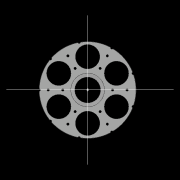
# Autodesk Inventor part: Top_Rotor_TSB
Saved by Autodesk Inventor 2022.2 (Build 262287010, 287A)
## iProperties
Created: 2022-05-21
Part Number: Top_Rotor_TSB
Material: Generic
Document SubType Name: Modeling
Designer: Árni Þór Þorgeirsson
Density: 1 g/cm^3
Appearance: Default
Author: Árni Þór Þorgeirsson
Autodesk Inventor part; units mm, degrees
ref_plane "YZ Plane" through (0, 0, 0) normal (1, 0, 0) x (0, 1, 0)
sketch "Sketch1" plane through (0, 0, 0) normal (0, 0, 1) x (1, 0, 0)
  circle A0 centre (0, 0) radius 13.3368 construction
  line L0 (0, 0) -> (13.3368, 0)
  line L1 (0, 0) -> (13.3368, 4.025)
  line L2 (13.3368, 0) -> (13.3368, 4.025)
  circle A1 centre (0, 0) radius 53.5
  dimension "d56" = 13.3368
  dimension "d57" = 4.025
  dimension "d400" = 53.5
  constraints: 6 end point, 2 coincident, 1 centre point, 1 horizontal, 1 horizontal alignment, 1 vertical, 6 other
  measures "d56" distance of L0.start L0.end
  measures "d57" distance of L1.end L0.end
  measures "d400" radius of A1
sketch "Sketch7" plane through (0, 0, 0) normal (0, 1, 0) x (-1, 0, 0)
  line L0 (0, 0) -> (0, 15.7673)
  line L1 (0, 0) -> (-13.3368, 0) construction
  line L2 (0, 15.7673) -> (-13.3368, 0) construction
  line L3 (0, 15.7673) -> (-18.6413, 0) construction
  line L4 (0, 15.7673) -> (-12.4569, -5.231) construction
  line L5 (0, 0) -> (0, -15.7673)
  line L6 (0, -15.7673) -> (-13.3368, 0) construction
  line L7 (0, -15.7673) -> (-18.6413, 0) construction
  line L8 (0, -15.7673) -> (-12.4569, 5.231) construction
  line L9 (-12.4569, 5.231) -> (-18.6413, 0) construction
  line L10 (-9.3537, 0) -> (-18.5948, -7.8164) construction
  line L11 (-9.3537, 0) -> (-18.0926, 7.3915) construction
  line L12 (0, -76.8701) -> (0, 74.6036) projected
  line L13 (-53.5, -5.9919) -> (-53.5, 6.008)
  line L14 (104.1947, 0) -> (-109.4074, 0) projected
  line L15 (-15.989, 2.2434) -> (-10.6846, -2.2434) construction
  line L16 (-10.6846, 2.2434) -> (-15.989, -2.2434) construction
  line L17 (-26.151, -15.9303) -> (-40.3783, -15.9303) construction
  line L18 (-40.3783, -15.9303) -> (-40.3783, -12.7539) construction
  line L19 (-40.3783, -12.7539) -> (-26.151, -12.7539) construction
  line L20 (-26.151, -12.7539) -> (-26.151, -15.9303) construction
  point P0 (-53.5, 0)
  dimension "Roller_Side_difference" = -0.0003
  dimension "d90" = 15.7673
  dimension "d201" = 53.5
  dimension "d343" = 99.548
  dimension "d344" = 99.549
  dimension "d367" = 8.1
  constraints: 28 end point, 9 point on line, 3 midpoint, 3 vertical, 2 horizontal, 2 parallel, 2 perpendicular, 1 collinear, 1 symmetric about line, 2 other
  measures "d90" distance of L0.start L0.end
  measures "d201" distance between parallel lines of L5 L13
  measures "d343" angle of L10 L8
  measures "d344" angle of L7 L10
  measures "d367" distance of L3.end L8.end
sketch "Roller1" plane through (0, 0, 0) normal (0, 1, 0) x (-1, 0, 0)
  line L0 (0, 15.7673) -> (-12.4569, -5.231) construction
  line L1 (0, 15.7673) -> (-18.6413, 0) construction
  line L2 (-9.3537, 0) -> (-18.0926, 7.3915) construction
  line L3 (0, -15.7673) -> (-18.6413, 0) construction
  line L4 (-9.4248, -0.0708) -> (-12.4245, -5.1274)
  line L5 (-12.4245, -5.1274) -> (-18.5445, 0.0491)
  line L6 (-18.5445, 0.0491) -> (-14.0556, 3.846)
  line L7 (-14.0556, 3.846) -> (-9.4248, -0.0708)
  line L8 (-11.7456, 1.8921) -> (-15.4898, -2.5346)
  line L9 (-10.9821, 1.2463) -> (-14.7263, -3.1804)
  point P0 (0, 0)
  point P1 (-15.4845, -2.5391)
  dimension "d345" = 0.025
  dimension "d346" = 0.025
  dimension "d347" = 0.1
  dimension "d348" = 0.1
  dimension "d349" = 99.549
  dimension "d350" = 99.548
  dimension "d357" = 1
  dimension "d369" = 4.0148
  constraints: 12 end point, 5 parallel, 4 point on line, 1 midpoint, 1 perpendicular
  measures "d345" distance between parallel lines of L0 L4
  measures "d346" distance between parallel lines of L1 L6
  measures "d347" distance between parallel lines of L3 L5
  measures "d348" distance between parallel lines of L2 L7
  measures "d349" angle of L6 L7
  measures "d350" angle of L4 L7
  measures "d357" distance between parallel lines of L8 L9
  measures "d369" distance from line of L4.end L8
sketch "Roller2" plane through (0, 0, 0) normal (0, 1, 0) x (-1, 0, 0)
  line L0 (0, -15.7673) -> (-12.4569, 5.231) construction
  line L1 (-9.3537, 0) -> (-18.5948, -7.8164) construction
  line L2 (0, -15.7673) -> (-18.6413, 0) construction
  line L3 (0, 15.7673) -> (-18.6413, 0) construction
  line L4 (-12.4633, 5.1928) -> (-9.386, 0.0054)
  line L5 (-9.386, 0.0054) -> (-13.9975, -3.8951)
  line L6 (-13.9975, -3.8951) -> (-18.6026, 0)
  line L7 (-18.6026, 0) -> (-12.4633, 5.1928)
  line L8 (-15.533, 2.5964) -> (-11.6918, -1.9449)
  line L9 (-14.7694, 3.2422) -> (-10.9283, -1.2991)
  point P0 (0, 0)
  dimension "d351" = 0.025
  dimension "d352" = 0.025
  dimension "d354" = 0.025
  dimension "d355" = 99.548
  dimension "d356" = 99.549
  dimension "d370" = 0.025
  dimension "d371" = 1
  constraints: 12 end point, 5 parallel, 3 point on line, 1 midpoint, 1 perpendicular
  measures "d351" distance between parallel lines of L0 L4
  measures "d352" distance between parallel lines of L2 L6
  measures "d354" distance between parallel lines of L1 L5
  measures "d355" angle of L5 L4
  measures "d356" angle of L6 L5
  measures "d370" distance from line of L3 L8.start
  measures "d371" distance between parallel lines of L9 L8
sketch "Sketch22" plane through (0, 0, 0) normal (0, 1, 0) x (-1, 0, 0)
  line L0 (-31.756, 8.0215) -> (-17.5287, 8.0215) construction
  line L1 (-17.5287, 8.0215) -> (-17.5287, 4.8451) construction
  line L2 (-17.5287, 4.8451) -> (-31.756, 4.8451) construction
  line L3 (-31.756, 4.8451) -> (-31.756, 8.0215) construction
  point P0 (0, 0)
  dimension "Roller_Side_difference" = -0.0003
  constraints: 2 other
sketch "Sketch2" plane through (0, 0, 0) normal (0, 1, 0) x (-1, 0, 0)
  line L0 (0, 0) -> (0, 13.3368) construction
  line L1 (0, 0) -> (-13.3368, 0) projected
  line L2 (0, 0) -> (0, -13.3368)
  line L3 (0, -13.3368) -> (-13.3368, 0) construction
  line L4 (0, 13.3368) -> (-13.3368, 0) construction
  line L5 (-78.8928, 52.9645) -> (0, 13.3368) construction
  line L6 (-34.8011, 15.91) -> (0, 13.3368) construction
  line L7 (-34.8011, 15.91) -> (0, -13.3368) construction
  line L8 (-48.3339, 16.9106) -> (0, -13.3368) construction
  point P0 (-17.4708, -4.134)
  constraints: 16 end point, 3 point on line, 1 perpendicular, 1 symmetric about line, 1 vertical
sketch "Sketch23" plane through (0, 0, 0) normal (0, 1, 0) x (-1, 0, 0)
  line L0 (0, -15.7673) -> (-12.4569, 5.231) construction
  line L1 (0, -15.7673) -> (-18.6413, 0) construction
  line L2 (0, 15.7673) -> (-12.4569, -5.231) construction
  line L3 (-12.4569, 5.231) -> (-18.6413, 0) construction
  line L4 (0, 15.7673) -> (-18.6413, 0) construction
  line L5 (-12.4569, 5.231) -> (-12.4569, -5.231) construction
  line L6 (104.1947, 0) -> (-109.4074, 0) projected
  line L7 (-11.538, 3.731) -> (-9.3549, 0.051)
  line L8 (-9.3549, -0.051) -> (-11.538, -3.731)
  line L9 (-14.269, 3.731) -> (-18.5898, 0.0764)
  line L10 (-18.5898, -0.0764) -> (-14.269, -3.731)
  arc A0 (-18.5898, 0.0764) -> (-18.5898, -0.0764) centre (-18.5252, 0) ccw
  arc A1 (-9.3549, -0.051) -> (-9.3549, 0.051) centre (-9.4409, 0) ccw
  line L11 (-11.538, 3.731) -> (-11.538, 5.231)
  line L12 (-11.538, 5.231) -> (-1, 5.231)
  line L13 (-1, 5.231) -> (-1, -5.231)
  line L14 (-1, -5.231) -> (-11.538, -5.231)
  line L15 (-11.538, -5.231) -> (-11.538, -3.731)
  line L16 (-14.269, 3.731) -> (-14.269, 5.231)
  line L17 (-14.269, 5.231) -> (-53.5, 5.231)
  line L18 (-53.5, 5.231) -> (-53.5, -5.231)
  line L19 (-14.269, -3.731) -> (-14.269, -5.231)
  line L20 (-14.269, -5.231) -> (-53.5, -5.231)
  line L21 (-12.4569, 5.231) -> (-12.4569, 5.231)
  line L22 (-12.4569, -5.231) -> (-12.4569, -5.231)
  line L23 (0, -76.8701) -> (0, 74.6036) projected
  line L24 (-18.68, 0) -> (-53.5, 0)
  point P0 (0, 0)
  point P1 (-9.3246, 0)
  point P2 (-18.6252, 0)
  point P3 (-53.5, 0)
  dimension "d378" = 90
  dimension "d379" = 0.1
  dimension "d380" = 0.025
  dimension "d381" = 0.025
  dimension "d382" = 0.025
  dimension "d383" = 0.025
  dimension "d384" = 10.4619
  dimension "d385" = 0
  dimension "d386" = 0
  dimension "d391" = 1
  dimension "d392" = 53.5
  dimension "d393" = 1.5
  dimension "d394" = 1.5
  dimension "d395" = 1.5
  dimension "d396" = 1.5
  constraints: 36 end point, 10 point on line, 9 vertical, 4 horizontal, 4 parallel, 4 point on circle, 4 tangent, 2 centre point, 1 equal radius, 1 midpoint
  measures "d378" angle of L6 L5
  measures "d379" radius of A0
  measures "d380" distance between parallel lines of L9 L4
  measures "d381" distance between parallel lines of L10 L1
  measures "d382" distance between parallel lines of L0 L7
  measures "d383" distance between parallel lines of L2 L8
  measures "d384" distance of L0.end L2.end
  measures "d385" distance of L2.end L22.end
  measures "d386" distance of L0.end L21.end
  measures "d391" distance between parallel lines of L23 L13
  measures "d392" distance between parallel lines of L18 L23
  measures "d393" distance of L9.start L16.end
  measures "d394" distance of L7.start L11.end
  measures "d395" distance of L14.end L8.end
  measures "d396" distance of L10.end L19.end
revolve "RevRoller1" [suppressed]
fillet "Fillet1" [suppressed]
pattern_circular "Circular Pattern13" [suppressed]
feature "Move Body7" [suppressed]
revolve "Revolution13" [suppressed]
fillet "Fillet3" [suppressed]
pattern_circular "Circular Pattern14" [suppressed]
feature "Move Body6" [suppressed]
revolve "Revolution14" [suppressed]
revolve "OuterRim_Top2" add sketch "Sketch23" angle 360 about axis through (0, 0, -10) along (0, 0, 1) contours L6 A0 L10 L19 L20 L18
revolve "OuterRim_Bottom2" [suppressed]
extrude "Rotor_Ring" [suppressed]
draft "FaceDraft2" angle 2.5 pull direction (0, 0, 1) faces at (-39.8716, -35.6721, -1.7437) fixed edges at (-53.5, 0, -5.231)
sketch "Sketch30" plane through (0, 0, 5.231) normal (0, 0, 1) x (1, 0, 0)
  circle A0 centre (0, 0) radius 1 projected
  line L0 (0, 0) -> (2.5, 0)
  circle A1 centre (2.5, 0) radius 4
  dimension "d495" = 2.5
  dimension "d496" = 8
  constraints: 2 end point, 1 centre point, 1 coincident, 1 horizontal
  measures "d495" distance of L0.start L0.end
  measures "d496" diameter of A1
ref_plane "Work Plane5" through (0, 0, 50) normal (0, 0, 1) x (1, 0, 0)
sketch "Rotor Featurs" plane through (0, 0, 50) normal (0, 0, 1) x (1, 0, 0)
  circle A0 centre (0, 0) radius 53.5 projected
  circle A1 centre (0, 0) radius 14.269 projected
  circle A2 centre (0, 0) radius 1 projected
  circle A3 centre (0, 0) radius 43.5
  circle A4 centre (0, 0) radius 36.75
  circle A5 centre (0, 0) radius 27.5
  line L0 (-56.25, 1.5877) -> (-53.5, 3.1754)
  line L1 (-53.5, 3.1754) -> (-50.75, 1.5877)
  line L2 (-50.75, 1.5877) -> (-50.75, -1.5877)
  line L3 (-50.75, -1.5877) -> (-53.5, -3.1754)
  line L4 (-53.5, -3.1754) -> (-56.25, -1.5877)
  line L5 (-56.25, -1.5877) -> (-56.25, 1.5877)
  line L6 (-40.75, -1.5877) -> (-43.5, -3.1754)
  line L7 (-43.5, -3.1754) -> (-46.25, -1.5877)
  line L8 (-46.25, -1.5877) -> (-46.25, 1.5877)
  line L9 (-46.25, 1.5877) -> (-43.5, 3.1754)
  line L10 (-43.5, 3.1754) -> (-40.75, 1.5877)
  line L11 (-40.75, 1.5877) -> (-40.75, -1.5877)
  line L12 (-30.25, 1.5877) -> (-27.5, 3.1754)
  line L13 (-27.5, 3.1754) -> (-24.75, 1.5877)
  line L14 (-24.75, 1.5877) -> (-24.75, -1.5877)
  line L15 (-24.75, -1.5877) -> (-27.5, -3.1754)
  line L16 (-27.5, -3.1754) -> (-30.25, -1.5877)
  line L17 (-30.25, -1.5877) -> (-30.25, 1.5877)
  circle A6 centre (-31.8264, -18.375) radius 13.5
  circle A7 centre (-53.5, 0) radius 1.5
  circle A8 centre (-53.5, 0) radius 2.75
  circle A9 centre (-43.5, 0) radius 1.5
  circle A10 centre (-27.5, 0) radius 1.5
  circle A11 centre (-43.5, 0) radius 2.75
  circle A12 centre (-27.5, 0) radius 2.75
  line L18 (-11.6213, -17.5209) -> (20.5249, -17.5209) construction
  line L19 (20.5249, -17.5209) -> (20.5249, -24.7583) construction
  line L20 (20.5249, -24.7583) -> (-11.6213, -24.7583) construction
  line L21 (-11.6213, -24.7583) -> (-11.6213, -17.5209) construction
  circle A13 centre (0, 0) radius 18.6252 projected
  line L22 (-56.25, 7.1754) -> (-50.75, 7.1754)
  line L23 (-50.75, 7.1754) -> (-50.75, 6.1754)
  line L24 (-50.75, 6.1754) -> (-56.25, 6.1754)
  line L25 (-56.25, 6.1754) -> (-56.25, 7.1754)
  line L26 (-56.25, -7.1754) -> (-56.25, -6.1754)
  line L27 (-56.25, -6.1754) -> (-50.75, -6.1754)
  line L28 (-50.75, -7.1754) -> (-56.25, -7.1754)
  line L29 (-50.75, -6.1754) -> (-50.75, -7.1754)
  point P0 (-56.25, -1.5877)
  point P1 (-50.75, -1.5877)
  dimension "d534" = 87
  dimension "d535" = 73.5
  dimension "d536" = 55
  dimension "Bearing_Roller_Gap_Reduction" = 0.3
  dimension "d531" = 5.5
  dimension "d532" = 5.5
  dimension "d533" = 5.5
  dimension "d537" = 27
  dimension "d538" = 3
  dimension "d543" = 5.5
  dimension "d549" = 3
  dimension "d550" = 3
  dimension "d567" = 5.5
  dimension "d568" = 5.5
  dimension "d617" = 1
  dimension "d618" = 3
  dimension "d621" = 360
  constraints: 52 end point, 12 coincident, 7 centre point, 4 point on line, 3 horizontal alignment, 2 parallel, 1 collinear, 1 horizontal, 1 perpendicular, 70 other
  measures "d531" distance between parallel lines of L5 L2
  measures "d532" distance between parallel lines of L11 L8
  measures "d533" distance between parallel lines of L17 L14
  measures "d537" diameter of A6
  measures "d538" diameter of A7
  measures "d543" diameter of A8
  measures "d549" diameter of A9
  measures "d550" diameter of A10
  measures "d567" diameter of A11
  measures "d568" diameter of A12
  measures "d617" distance of L22.end L23.end
  measures "d618" distance from line of L24 L0.end
sketch "RotorRim_Bottom" plane through (0, 0, 5.231) normal (0, 0, 1) x (1, 0, 0)
  line L0 (-53.5, 3.1754) -> (-50.75, 1.5877) projected
  line L1 (-56.25, 1.5877) -> (-53.5, 3.1754) projected
  line L2 (-56.25, -1.5877) -> (-56.25, 1.5877) projected
  line L3 (-53.5, -3.1754) -> (-56.25, -1.5877) projected
  line L4 (-50.75, -1.5877) -> (-53.5, -3.1754) projected
  circle A0 centre (0, 0) radius 53.5 projected
  circle A1 centre (-53.5, 0) radius 1.5 projected
  point P0 (-53.4088, 3.1228)
  point P1 (-53.4088, -3.1228)
  point P2 (-53.479, -1.4999)
  point P3 (-53.479, 1.4999)
  constraints: 1 other
extrude "Extrusion24" [suppressed]
extrude "Extrusion25" [suppressed]
sketch "Sketch40" plane through (0, 0, -5.231) normal (0, 0, -1) x (-1, 0, 0)
  circle A0 centre (53.5, 0) radius 2.75 projected
  circle A1 centre (0, 0) radius 53.5 projected
  point P0 (53.4293, 2.7491)
  point P1 (53.4293, -2.7491)
extrude "Extrusion26" [suppressed]
pattern_circular "Circular Pattern23" [suppressed]
sketch "Sketch41" plane through (0, 0, 5.231) normal (0, 0, 1) x (1, 0, 0)
  circle A0 centre (0, 0) radius 53.5 projected
  circle A1 centre (-53.5, 0) radius 1.5 projected
  circle A2 centre (-43.5, 0) radius 1.5 projected
  circle A3 centre (-27.5, 0) radius 1.5 projected
  line L0 (-53.5, 3.1754) -> (-50.75, 1.5877) projected
  line L1 (-50.75, 1.5877) -> (-50.75, -1.5877) projected
  line L2 (-50.75, -1.5877) -> (-53.5, -3.1754) projected
  line L3 (-46.25, 1.5877) -> (-43.5, 3.1754) projected
  line L4 (-46.25, -1.5877) -> (-46.25, 1.5877) projected
  line L5 (-43.5, -3.1754) -> (-46.25, -1.5877) projected
  line L6 (-40.75, -1.5877) -> (-43.5, -3.1754) projected
  line L7 (-40.75, 1.5877) -> (-40.75, -1.5877) projected
  line L8 (-43.5, 3.1754) -> (-40.75, 1.5877) projected
  line L9 (-30.25, 1.5877) -> (-27.5, 3.1754) projected
  line L10 (-30.25, -1.5877) -> (-30.25, 1.5877) projected
  line L11 (-27.5, -3.1754) -> (-30.25, -1.5877) projected
  line L12 (-24.75, -1.5877) -> (-27.5, -3.1754) projected
  line L13 (-24.75, 1.5877) -> (-24.75, -1.5877) projected
  line L14 (-27.5, 3.1754) -> (-24.75, 1.5877) projected
  circle A4 centre (-31.8264, -18.375) radius 13.5 projected
  point P0 (-53.4088, -3.1228)
  point P1 (-53.4088, 3.1228)
  point P2 (-53.479, 1.4999)
  point P3 (-53.479, -1.4999)
extrude "Extrusion27" [suppressed]
extrude "Extrusion28" [suppressed]
pattern_circular "Circular Pattern24" [suppressed]
extrude "Extrusion29" [suppressed]
extrude "Extrusion30" [suppressed]
extrude "Extrusion31" [suppressed]
pattern_of_nothing "Circular Pattern25"
sketch "Sketch42" plane through (0, 0, -5.231) normal (0, 0, -1) x (-1, 0, 0)
  circle A0 centre (53.5, 0) radius 2.75 projected
  circle A1 centre (0, 0) radius 53.5 projected
  circle A2 centre (43.5, 0) radius 2.75 projected
  circle A3 centre (27.5, 0) radius 2.75 projected
  circle A4 centre (53.5, 0) radius 1.5 projected
  circle A5 centre (43.5, 0) radius 1.5 projected
  circle A6 centre (27.5, 0) radius 1.5 projected
  circle A7 centre (31.8264, -18.375) radius 13.5 projected
  point P0 (53.4293, 2.7491)
  point P1 (53.4293, -2.7491)
  point P2 (53.479, 1.4999)
  point P3 (53.479, -1.4999)
extrude "Extrusion32" cut sketch "Sketch42" against normal blind 3 contours A1 A4 A0 | A1 A4 picked at (51.1832, -0.0597) picked at (53.0311, 0.3425)
extrude "Extrusion33" cut sketch "Sketch42" against normal blind 5.231 contours A1 A4 picked at (53.0311, 0.3425)
extrude "Extrusion34" cut sketch "Sketch42" against normal blind 3 contours A2 | A3 | A5 | A6
extrude "Extrusion35" cut sketch "Sketch42" against normal blind 5.231 contours A5 | A6 | A7
pattern_circular "Circular Pattern26" count 9 over 360 about axis through (0, 0, -10) along (0, 0, 1) of "Extrusion32", "Extrusion33"
pattern_circular "Circular Pattern27" count 6 over 360 about axis through (0, 0, -10) along (0, 0, 1) of "Extrusion34", "Extrusion35"
chamfer "Chamfer1" [suppressed]
chamfer "Chamfer2" [suppressed]
feature "FaceDraft4" [suppressed]
ref_plane "Work Plane7" through (-0.5825, 0.0099, -55.231) normal (0, 0, -1) x (-1, 0, 0)
sketch "Sketch44" plane through (-0.5825, 0.0099, -55.231) normal (0, 0, -1) x (-1, 0, 0)
  point P0 (58.7175, -0.0099)
sketch "Sketch45" plane through (0, 0, 50) normal (0, 0, 1) x (1, 0, 0)
  point P0 (-51.8, 0)
extrude "Extrusion39" cut sketch "Rotor Featurs" along normal blind 0.8 from surface at -55.231 contours L22 L23 L24 A0 | A0 L24 L25 L22 | L28 L26 L27 A0 | A0 L27 L29 L28
extrude "Extrusion40" [suppressed]
ref_plane "Work Plane8" through (0, 0, 20) normal (0, 0, 1) x (1, 0, 0)
sketch "Sketch46" plane through (0, 0, 20) normal (0, 0, 1) x (1, 0, 0)
  spline S0 degree 3 poles (56.8, 0) (56.8, -1.4319) (57.0266, -2.8218) (57.3141, -4.0377) (57.7676, -5.9558) (58.3249, -7.5697) (58.7222, -9.3953) (59.1369, -11.3012) (59.3869, -13.435) (59.2247, -15.7235) (59.0417, -18.3045) (58.3019, -21.0371) (57.0692, -23.4317) (55.9716, -25.5639) (54.5147, -27.4028) (52.9916, -28.8594) (51.6098, -30.1808) (50.1991, -31.1871) (48.7772, -32.1565) (47.6582, -32.9193) (46.4886, -33.6761) (45.2876, -34.7145) (44.2461, -35.6149) (43.2239, -36.7614) (42.4465, -37.9481) (41.5522, -39.3132) (40.9615, -40.6395) (40.4023, -41.8816) (39.6981, -43.4458) (39.012, -44.9714) (38.0364, -46.5419) (36.8523, -48.4481) (35.229, -50.3909) (33.1724, -51.9911) (31.0828, -53.6171) (28.5762, -54.8431) (26.0987, -55.5082) (23.9667, -56.0805) (21.8887, -56.2534) (19.9964, -56.2163) (18.2263, -56.1816) (16.6275, -55.9648) (14.8704, -55.8135) (13.6437, -55.7079) (12.287, -55.6403) (10.8418, -55.7977) (9.4051, -55.954) (7.9582, -56.3561) (6.723, -56.8409) (4.72, -57.6271) (3.1609, -58.5239) (1.3743, -59.2859) (-0.4339, -60.0571) (-2.4841, -60.7211) (-4.7859, -61.008) (-7.2974, -61.3212) (-10.0699, -61.1458) (-12.6364, -60.4279) (-15.0685, -59.7477) (-17.2767, -58.6047) (-19.0781, -57.3063) (-20.675, -56.1553) (-21.9478, -54.9116) (-23.1791, -53.6504) (-24.0931, -52.7142) (-25.0062, -51.7331) (-26.1738, -50.758) (-27.2513, -49.8582) (-28.5815, -49.0078) (-29.9203, -48.4225) (-31.362, -47.7921) (-32.7293, -47.438) (-34.0061, -47.1128) (-35.7099, -46.6787) (-37.3575, -46.2745) (-39.1066, -45.5849) (-41.1221, -44.7903) (-43.2458, -43.605) (-45.1448, -41.9571) (-47.1257, -40.238) (-48.8124, -38.0317) (-49.9482, -35.7294) (-50.9787, -33.6408) (-51.5623, -31.5143) (-51.8755, -29.5515) (-52.1638, -27.7446) (-52.2245, -26.087) (-52.3894, -24.2693) (-52.5001, -23.0492) (-52.6748, -21.7055) (-53.0824, -20.3178) (-53.486, -18.9435) (-54.1251, -17.6047) (-54.8078, -16.4847) (-55.8849, -14.7175) (-56.9946, -13.3786) (-58.0206, -11.8296) (-59.0577, -10.2638) (-60.0421, -8.4781) (-60.746, -6.3918) (-61.5632, -3.97) (-61.9524, -1.1678) (-61.7393, 1.5511) (-61.5477, 3.9947) (-60.8853, 6.3317) (-59.9849, 8.3224) (-59.1769, 10.1091) (-58.2036, 11.607) (-57.2044, 13.0158) (-56.3467, 14.2251) (-55.4319, 15.3943) (-54.5714, 16.8827) (-53.8946, 18.0531) (-53.296, 19.4496) (-52.9414, 20.8302) (-52.5526, 22.3437) (-52.4247, 23.7538) (-52.324, 25.055) (-52.1844, 26.8594) (-52.0852, 28.5763) (-51.715, 30.453) (-51.2878, 32.618) (-50.4834, 34.9703) (-49.1585, 37.1767) (-47.7999, 39.439) (-45.9031, 41.4933) (-43.8164, 43.0144) (-41.9871, 44.3479) (-40.05, 45.273) (-38.2187, 45.9151) (-36.4508, 46.5351) (-34.7962, 46.8888) (-33.0011, 47.3754) (-31.816, 47.6967) (-30.5213, 48.102) (-29.2246, 48.7472) (-27.9361, 49.3883) (-26.7251, 50.2594) (-25.7377, 51.1332) (-24.1248, 52.5605) (-22.9654, 53.9373) (-21.5425, 55.266) (-20.1382, 56.5772) (-18.4817, 57.8699) (-16.4757, 58.9115) (-14.1658, 60.1108) (-11.4118, 60.9217) (-8.673, 61.1141) (-6.2167, 61.2866) (-3.8151, 60.9744) (-1.7249, 60.3891) (0.129, 59.87) (1.7254, 59.1596) (3.276, 58.4164) (4.5061, 57.8267) (5.74, 57.1881) (7.2319, 56.649) (8.5094, 56.1873) (9.9929, 55.8479) (11.4103, 55.7465) (12.9863, 55.6336) (14.4057, 55.7628) (15.7204, 55.893) (17.5126, 56.0705) (19.2283, 56.2635) (21.1474, 56.213) (23.3514, 56.155) (25.8006, 55.7542) (28.1882, 54.8225) (30.6413, 53.8653) (32.9754, 52.3479) (34.8186, 50.5592) (36.4742, 48.9526) (37.7272, 47.1676) (38.6791, 45.4442) (39.6023, 43.7728) (40.2354, 42.1708) (41.0732, 40.4265) (41.6043, 39.3209) (42.257, 38.119) (43.1325, 36.9822) (43.9863, 35.8733) (45.0213, 34.896) (46.0149, 34.1163) (47.6582, 32.827) (49.1789, 31.938) (50.7017, 30.7916) (52.2598, 29.6185) (53.8446, 28.1841) (55.2311, 26.3515) (56.7985, 24.28) (58.0545, 21.7118) (58.7031, 19.0595) (59.2916, 16.6532) (59.3854, 14.2226) (59.1574, 12.0576) (58.9571, 10.1553) (58.5292, 8.4737) (58.0655, 6.8215) (57.7157, 5.5753) (57.3275, 4.3132) (57.063, 2.8386) (56.9031, 1.9472) (56.8, 0.9776) (56.8, 0) knots 0 0 0 0 3.630189 3.630189 3.630189 9.356968 9.356968 9.356968 15.335248 15.335248 15.335248 22.077576 22.077576 22.077576 28.081487 28.081487 28.081487 33.527934 33.527934 33.527934 37.813991 37.813991 37.813991 41.530754 41.530754 41.530754 45.806559 45.806559 45.806559 51.191166 51.191166 51.191166 57.726747 57.726747 57.726747 64.367473 64.367473 64.367473 70.081985 70.081985 70.081985 75.427611 75.427611 75.427611 79.15967 79.15967 79.15967 82.86972 82.86972 82.86972 88.885508 88.885508 88.885508 94.974003 94.974003 94.974003 101.617247 101.617247 101.617247 107.912495 107.912495 107.912495 113.492866 113.492866 113.492866 117.63499 117.63499 117.63499 121.457377 121.457377 121.457377 125.573774 125.573774 125.573774 131.06692 131.06692 131.06692 137.396362 137.396362 137.396362 143.99916 143.99916 143.99916 149.989436 149.989436 149.989436 155.503632 155.503632 155.503632 159.204798 159.204798 159.204798 162.870082 162.870082 162.870082 168.653221 168.653221 168.653221 174.498759 174.498759 174.498759 181.284424 181.284424 181.284424 187.383433 187.383433 187.383433 192.857431 192.857431 192.857431 197.5563 197.5563 197.5563 201.251307 201.251307 201.251307 205.301831 205.301831 205.301831 210.91873 210.91873 210.91873 217.398706 217.398706 217.398706 224.043346 224.043346 224.043346 229.86837 229.86837 229.86837 235.491984 235.491984 235.491984 239.204835 239.204835 239.204835 242.894294 242.894294 242.894294 248.920758 248.920758 248.920758 254.86843 254.86843 254.86843 261.717359 261.717359 261.717359 267.860024 267.860024 267.860024 273.30815 273.30815 273.30815 277.630663 277.630663 277.630663 281.332185 281.332185 281.332185 285.447681 285.447681 285.447681 291.057972 291.057972 291.057972 297.50109 297.50109 297.50109 304.120892 304.120892 304.120892 310.066772 310.066772 310.066772 315.832644 315.832644 315.832644 319.487459 319.487459 319.487459 323.052251 323.052251 323.052251 328.947474 328.947474 328.947474 334.97976 334.97976 334.97976 341.798889 341.798889 341.798889 347.985491 347.985491 347.985491 353.421408 353.421408 353.421408 357.521549 357.521549 357.521549 360 360 360 360 projected
  circle A0 centre (62.6801, -0.0744) radius 6
  line L0 (0, 0) -> (-2.5, 0)
  circle A1 centre (50.2755, 38.2517) radius 6
  circle A2 centre (17.7125, 61.9669) radius 6
  circle A3 centre (-22.571, 62.0129) radius 6
  circle A4 centre (-55.1881, 38.3721) radius 6
  circle A5 centre (-67.6801, 0.0744) radius 6
  circle A6 centre (-55.2755, -38.2517) radius 6
  circle A7 centre (-22.7125, -61.9669) radius 6
  circle A8 centre (17.571, -62.0129) radius 6
  circle A9 centre (50.1881, -38.3721) radius 6
  spline S1 degree 3 poles (56.8, 0) (56.8, -1.327) (57.0234, -2.6109) (57.3007, -3.6923) (57.7543, -5.4607) (58.2895, -6.8218) (58.7112, -8.3283) (59.1721, -9.9753) (59.5267, -11.7944) (59.5593, -13.8117) (59.598, -16.208) (59.1382, -18.8439) (58.1536, -21.2237) (57.2965, -23.2955) (56.0684, -25.1435) (54.7369, -26.6222) (53.5473, -27.9433) (52.3032, -28.9676) (51.052, -29.9022) (50.046, -30.6537) (49.006, -31.3468) (47.8554, -32.3233) (46.9843, -33.0626) (46.0484, -34.0152) (45.2938, -35.1119) (44.5396, -36.2079) (44.0054, -37.3704) (43.6138, -38.3974) (42.983, -40.052) (42.6128, -41.4454) (42.0619, -42.8993) (41.4492, -44.516) (40.6333, -46.2151) (39.4339, -47.8713) (38.032, -49.8072) (36.0969, -51.6271) (33.9087, -52.9343) (31.9495, -54.1046) (29.8285, -54.8554) (27.8576, -55.2437) (26.1429, -55.5815) (24.5642, -55.6603) (23.0139, -55.6752) (21.7466, -55.6873) (20.4668, -55.6358) (18.9158, -55.7787) (17.7446, -55.8866) (16.399, -56.1544) (15.1593, -56.6349) (13.9089, -57.1195) (12.8329, -57.7662) (11.9323, -58.3732) (10.4683, -59.3599) (9.3245, -60.279) (7.9625, -61.1406) (6.4559, -62.0937) (4.6989, -62.9801) (2.6661, -63.5673) (0.3544, -64.235) (-2.2833, -64.4684) (-4.7798, -64.1594) (-7.0414, -63.8794) (-9.1504, -63.1755) (-10.9222, -62.2948) (-12.4361, -61.5424) (-13.6962, -60.6844) (-14.941, -59.7881) (-15.9425, -59.067) (-16.9561, -58.2795) (-18.3098, -57.5157) (-19.3549, -56.926) (-20.6338, -56.3928) (-21.9035, -56.0972) (-23.2354, -55.7871) (-24.4767, -55.715) (-25.5637, -55.6914) (-27.252, -55.6547) (-28.7024, -55.7096) (-30.3012, -55.5868) (-32.1878, -55.4419) (-34.2662, -55.0517) (-36.3567, -54.2041) (-38.6022, -53.2938) (-40.805, -51.844) (-42.5524, -50.0858) (-44.1477, -48.4804) (-45.35, -46.659) (-46.1982, -44.9141) (-46.94, -43.3878) (-47.4157, -41.9455) (-47.9119, -40.4276) (-48.2662, -39.3437) (-48.6345, -38.1705) (-49.2732, -36.8659) (-49.8415, -35.7053) (-50.6735, -34.4812) (-51.5908, -33.5134) (-52.5793, -32.4705) (-53.5785, -31.7191) (-54.4815, -31.054) (-55.7719, -30.1035) (-56.9658, -29.2673) (-58.1708, -28.1834) (-59.6101, -26.8888) (-61.0408, -25.2456) (-62.1667, -23.2509) (-63.4169, -21.0357) (-64.2365, -18.4173) (-64.477, -15.9) (-64.6864, -13.708) (-64.4799, -11.6321) (-64.0824, -9.8109) (-63.7377, -8.2319) (-63.2593, -6.8589) (-62.7733, -5.3187) (-62.4416, -4.2676) (-62.0874, -3.086) (-61.9088, -1.6884) (-61.7416, -0.3793) (-61.7884, 1.0779) (-62.0061, 2.3332) (-62.2809, 3.918) (-62.7245, 5.173) (-63.1084, 6.3618) (-63.5857, 7.8398) (-64.0285, 9.2882) (-64.3004, 10.9509) (-64.6311, 12.9738) (-64.6775, 15.2937) (-64.2284, 17.6343) (-63.7598, 20.0763) (-62.7437, 22.4881) (-61.4161, 24.469) (-60.332, 26.0866) (-59.0714, 27.4119) (-57.8129, 28.4988) (-56.5938, 29.5517) (-55.3903, 30.3668) (-54.0597, 31.3676) (-53.2039, 32.0113) (-52.2562, 32.7675) (-51.3507, 33.7733) (-50.4416, 34.783) (-49.6557, 36.0299) (-49.1234, 37.1808) (-48.4221, 38.6971) (-48.0555, 40.0041) (-47.6412, 41.2524) (-47.15, 42.7324) (-46.6064, 44.2048) (-45.7763, 45.7355) (-44.7411, 47.6446) (-43.2412, 49.6031) (-41.3334, 51.2075) (-39.4289, 52.809) (-37.1526, 54.0167) (-34.9373, 54.7142) (-33.1141, 55.2883) (-31.3598, 55.5342) (-29.7323, 55.6242) (-28.3513, 55.7006) (-27.0633, 55.6597) (-25.5864, 55.6909) (-24.5244, 55.7133) (-23.3181, 55.7804) (-22.0174, 56.0712) (-20.725, 56.3602) (-19.4113, 56.8974) (-18.3415, 57.4978) (-16.8985, 58.3079) (-15.8405, 59.1437) (-14.7779, 59.9053) (-13.4787, 60.8365) (-12.1375, 61.7296) (-10.5152, 62.4916) (-8.5819, 63.3996) (-6.2624, 64.0777) (-3.8277, 64.2524) (-1.4092, 64.426) (1.0769, 64.0915) (3.2393, 63.3918) (5.2098, 62.7542) (6.8896, 61.8487) (8.3517, 60.8899) (9.6525, 60.0367) (10.7724, 59.1259) (12.2575, 58.1575) (13.172, 57.5612) (14.2777, 56.9407) (15.5201, 56.5012) (16.758, 56.0632) (18.0589, 55.8429) (19.188, 55.7556) (21.0017, 55.6154) (22.449, 55.7036) (23.9664, 55.6569) (25.6247, 55.6058) (27.3882, 55.4279) (29.2594, 54.914) (31.4727, 54.3061) (33.7922, 53.1993) (35.775, 51.6589) (37.7092, 50.1563) (39.2871, 48.2756) (40.3989, 46.4009) (41.3078, 44.8682) (41.9163, 43.367) (42.4236, 41.8965) (42.8417, 40.6847) (43.181, 39.4701) (43.7474, 38.0554) (44.1655, 37.0111) (44.7518, 35.8353) (45.539, 34.7677) (46.3212, 33.7068) (47.2492, 32.8184) (48.1016, 32.1177) (49.5296, 30.9438) (50.7808, 30.1473) (52.0301, 29.1485) (53.4148, 28.0414) (54.8173, 26.7052) (56.0475, 24.9992) (57.4673, 23.0302) (58.596, 20.5803) (59.1411, 18.0619) (59.6321, 15.7931) (59.6558, 13.5141) (59.3835, 11.5063) (59.154, 9.8145) (58.7357, 8.3297) (58.2716, 6.8702) (57.9343, 5.8095) (57.5546, 4.7435) (57.2387, 3.4438) (56.9903, 2.422) (56.8, 1.2265) (56.8, 0) knots 0 0 0 0 2.92615 2.92615 2.92615 7.711434 7.711434 7.711434 12.943122 12.943122 12.943122 19.157864 19.157864 19.157864 24.568088 24.568088 24.568088 29.401756 29.401756 29.401756 33.288501 33.288501 33.288501 36.230894 36.230894 36.230894 39.171404 39.171404 39.171404 43.908512 43.908512 43.908512 49.175706 49.175706 49.175706 55.332579 55.332579 55.332579 60.844903 60.844903 60.844903 65.640655 65.640655 65.640655 69.561333 69.561333 69.561333 72.521926 72.521926 72.521926 75.507919 75.507919 75.507919 80.361628 80.361628 80.361628 85.730778 85.730778 85.730778 91.83639 91.83639 91.83639 97.367292 97.367292 97.367292 102.093013 102.093013 102.093013 105.895154 105.895154 105.895154 108.830703 108.830703 108.830703 111.909891 111.909891 111.909891 116.692427 116.692427 116.692427 122.335731 122.335731 122.335731 128.39751 128.39751 128.39751 133.932136 133.932136 133.932136 138.772975 138.772975 138.772975 142.229647 142.229647 142.229647 145.30473 145.30473 145.30473 148.618258 148.618258 148.618258 153.353675 153.353675 153.353675 159.009539 159.009539 159.009539 165.290491 165.290491 165.290491 170.759657 170.759657 170.759657 175.501694 175.501694 175.501694 178.738228 178.738228 178.738228 181.769664 181.769664 181.769664 185.596606 185.596606 185.596606 190.354215 190.354215 190.354215 196.143023 196.143023 196.143023 202.182649 202.182649 202.182649 207.114441 207.114441 207.114441 211.892115 211.892115 211.892115 214.965085 214.965085 214.965085 218.050084 218.050084 218.050084 222.114162 222.114162 222.114162 226.93272 226.93272 226.93272 232.942499 232.942499 232.942499 238.941668 238.941668 238.941668 243.878936 243.878936 243.878936 248.068708 248.068708 248.068708 251.081437 251.081437 251.081437 254.075144 254.075144 254.075144 258.11351 258.11351 258.11351 263.050833 263.050833 263.050833 268.934783 268.934783 268.934783 274.77958 274.77958 274.77958 280.105856 280.105856 280.105856 284.844835 284.844835 284.844835 287.762789 287.762789 287.762789 290.670157 290.670157 290.670157 295.340478 295.340478 295.340478 300.444349 300.444349 300.444349 306.481378 306.481378 306.481378 312.370067 312.370067 312.370067 317.184427 317.184427 317.184427 321.151584 321.151584 321.151584 324.080189 324.080189 324.080189 326.99017 326.99017 326.99017 331.865251 331.865251 331.865251 337.268391 337.268391 337.268391 343.504301 343.504301 343.504301 349.121972 349.121972 349.121972 353.855445 353.855445 353.855445 357.295493 357.295493 357.295493 360 360 360 360 projected
  point P0 (56.8, 0)
  dimension "d635" = 12
  dimension "d640" = 2.5
  dimension "d643" = 360
  dimension "d585" = 8
  dimension "d587" = 1.75
  dimension "d589" = 3
  dimension "d592" = 2
  dimension "d593" = 12
  dimension "d594" = 12
  dimension "d611" = 360
  constraints: 18 point on circle, 10 centre point, 8 end point, 2 midpoint, 1 horizontal alignment, 1 vertical, 29 other
  measures "d589" diameter of A1
equation "\"Roller_Side_difference\" = -0.001568deg"
equation "\"Bearing_Roller_Gap_Reduction\" = 0.3"
equation "\"Cycloid_Top_Plate_Fasner_Outer\" = 87"
equation "\"Roller_Hole_Radius\" = 1"
equation "\"Distance_To_Bearing\" = 20.65135"
equation "\"d514\" = 0.2"
body "Solid1"
body "Solid5"
